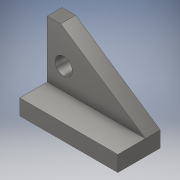
# Autodesk Inventor part: WoodenBlock
Saved by Autodesk Inventor 2019 (Build 230136000, 136)
## iProperties
Created: 2019-02-11
Part Number: WoodenBlock
Material: Stainless Steel
Document SubType Name: Modeling
Designer: Mihir
Density: 8 g/cm^3
Appearance: Semi-Polished
Mass: 589.768 g
Surface Area: 158.157 cm^2
Volume: 73.721 cm^3
Author: Mihir
Autodesk Inventor part; units mm, degrees
ref_plane "YZ Plane" through (0, 0, 0) normal (1, 0, 0) x (0, 1, 0)
ref_plane "XZ Plane" through (0, 0, 0) normal (0, 1, 0) x (-1, 0, 0)
ref_plane "XY Plane" through (0, 0, 0) normal (0, 0, 1) x (1, 0, 0)
sketch "Sketch1" plane through (0, 0, 0) normal (0, 0, 1) x (1, 0, 0)
  line L0 (0, 0) -> (0, 63.8302)
  line L1 (0, 63.8302) -> (11.8288, 63.8302)
  line L2 (11.8288, 63.8302) -> (86.0806, 13.7465)
  line L3 (86.0806, 13.7465) -> (86.0806, 0)
  line L4 (86.0806, 0) -> (0, 0)
  dimension "d0" = 11.8288
  dimension "d1" = 13.7465
  dimension "d2" = 63.8302
  dimension "d3" = 86.0806
  constraints: 10 end point, 2 perpendicular, 2 vertical
  measures "d0" distance of L0.end L1.end
  measures "d1" distance of L2.end L3.end
  measures "d2" distance of L0.start L0.end
  measures "d3" distance of L3.end L0.start
extrude "Extrusion1" add sketch "Sketch1" along normal blind 13.0607
sketch "Sketch3" plane through (0, 0, 13.0607) normal (0, 0, 1) x (1, 0, 0)
  line L0 (86.0806, 0) -> (86.0806, 13.7465) projected
  line L1 (86.0806, 13.7465) -> (0, 13.7465)
  line L2 (0, 13.7465) -> (0, 0)
  line L3 (0, 0) -> (86.0806, 0)
  line L4 (86.0806, 0) -> (86.0806, 13.7465)
  constraints: 8 end point, 2 parallel, 1 horizontal, 1 perpendicular
extrude "Extrusion2" add sketch "Sketch3" along normal blind 24.1529
sketch "Sketch4" plane through (0, 0, 13.0607) normal (0, 0, 1) x (1, 0, 0)
  circle A0 centre (14.478, 33.0708) radius 7.5463
  line L0 (11.8288, 63.8302) -> (0, 63.8302) projected
  line L1 (0, 63.8302) -> (0, 13.7465) projected
  point P0 (0, 0)
  dimension "d8" = 15.0927
  dimension "d9" = 30.7594
  dimension "d10" = 14.478
  constraints: 1 centre point
  measures "d8" diameter of A0
  measures "d9" distance from line of L0 A0.centre
  measures "d10" distance from line of L1 A0.centre
extrude "Extrusion3" cut sketch "Sketch4" against normal blind 24.1529
body "Solid1"
